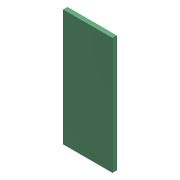
# Autodesk Inventor part: RJ45_PCB
Saved by Autodesk Inventor 2017 (Build 210142000, 142)
## iProperties
Created: 2017-11-20
Part Number: RJ45_PCB
Material: Generic
Document SubType Name: Modeling
Designer: Kathryn Rosie
Density: 1 g/cm^3
Appearance: Smooth - Dark Sea Green
Author: Kathryn Rosie
Autodesk Inventor part; units mm, degrees
ref_plane "YZ Plane" through (0, 0, 0) normal (1, 0, 0) x (0, 1, 0)
ref_plane "XZ Plane" through (0, 0, 0) normal (0, 1, 0) x (-1, 0, 0)
ref_plane "XY Plane" through (0, 0, 0) normal (0, 0, 1) x (1, 0, 0)
sketch "Sketch1" plane through (0, 0, 0) normal (0, 1, 0) x (-1, 0, 0)
  line L0 (-9.3, 21.975) -> (9.3, 21.975)
  line L1 (9.3, 21.975) -> (9.3, -21.975)
  line L2 (9.3, -21.975) -> (-9.3, -21.975)
  line L3 (-9.3, -21.975) -> (-9.3, 21.975)
  line L4 (-9.3, 21.975) -> (9.3, -21.975) construction
  line L5 (9.3, 21.975) -> (-9.3, -21.975) construction
  point P0 (0, 0)
  dimension "d0" = 43.95
  dimension "d1" = 18.6
  constraints: 12 end point, 2 midpoint, 2 parallel, 1 horizontal, 1 perpendicular
  measures "d0" distance of L0.end L1.end
  measures "d1" distance of L1.end L2.end
extrude "Extrusion1" add sketch "Sketch1" along normal blind 1.6
body "Solid1"
